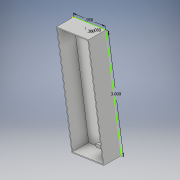
# Autodesk Inventor part: batteryHousing
Saved by Autodesk Inventor 2019.4 (Build 234330000, 330)
## iProperties
Created: 2019-10-21
Part Number: batteryHousing
Material: Generic
Document SubType Name: Modeling
Designer: nLaptop
Density: 1 g/cm^3
Appearance: Default
Author: nLaptop
Autodesk Inventor part; units mm, degrees
ref_plane "YZ Plane" through (0, 0, 0) normal (1, 0, 0) x (0, 1, 0)
ref_plane "XZ Plane" through (0, 0, 0) normal (0, 1, 0) x (-1, 0, 0)
ref_plane "XY Plane" through (0, 0, 0) normal (0, 0, 1) x (1, 0, 0)
sketch "Sketch1" plane through (0, 0, 0) normal (0, 0, 1) x (1, 0, 0)
  line L0 (0, 0) -> (23.8603, 3.5978)
  line L1 (23.8603, 3.5978) -> (35.2216, -71.7505)
  line L2 (35.2216, -71.7505) -> (11.3613, -75.3483)
  line L3 (11.3613, -75.3483) -> (0, 0)
  line L4 (12.1195, 0.5431) -> (15.8869, 1.1111)
  line L5 (15.8869, 1.1111) -> (16.1899, -0.8981)
  line L6 (16.1899, -0.8981) -> (8.6551, -2.0343)
  line L7 (8.6551, -2.0343) -> (8.3521, -0.025)
  line L8 (8.3521, -0.025) -> (12.1195, 0.5431)
  line L9 (23.1021, -72.2936) -> (26.8695, -71.7255)
  line L10 (26.8695, -71.7255) -> (26.5666, -69.7162)
  line L11 (26.5666, -69.7162) -> (19.0317, -70.8524)
  line L12 (19.0317, -70.8524) -> (19.3347, -72.8616)
  line L13 (19.3347, -72.8616) -> (23.1021, -72.2936)
  dimension "d0" = 24.13
  dimension "d1" = 76.2
  dimension "d9" = 2.032
  dimension "d10" = 7.62
  constraints: 28 end point, 9 perpendicular, 2 point on line
  measures "d0" distance of L0.start L0.end
  measures "d1" distance of L0.end L1.end
  measures "d9" distance of L4.end L5.end
  measures "d10" distance of L5.end L6.end
extrude "Extrusion1" add sketch "Sketch1" along normal blind 12.7 contours L0 L1 L2 L3 | L4 L5 L6 L7 L8 | L13 L12 L11 L10 L9
shell "Shell1" thickness 0.635 removed faces 1 at (23.4811, -47.8337, 12.7)
sketch "Sketch2" plane through (11.8946, -74.6257, 0.635) normal (0, 0, 1) x (0.9888, 0.1491, 0)
  point P0 (-0.635, 75.565)
extrude "Extrusion2" add sketch "Sketch1" along normal blind 2.54 contours L4 L5 L6 L7 L8 | L13 L12 L11 L10 L9
body "Solid1"
